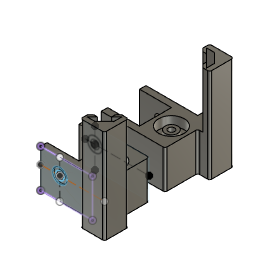
Bed Mount Lighted (Autodesk Fusion 360 design; units mm, degrees)
part number: Mount
Autodesk Fusion 360 part; units mm, degrees
sketch "Sketch1" plane through (0, 0, 0) normal (0, 0, 1) x (1, 0, 0) in component "Mount"
  line L0 (20, 14) -> (-20, 14)
  line L1 (-20, 14) -> (-20, -14)
  line L2 (-20, -14) -> (20, -14)
  line L3 (20, -14) -> (20, 14)
  line L4 (20, 14) -> (-20, -14) construction
  line L5 (-20, 14) -> (20, -14) construction
  line L6 (27.5, -6.5) -> (12.5, -6.5)
  line L7 (12.5, -6.5) -> (12.5, -21.5)
  line L8 (12.5, -21.5) -> (27.5, -21.5)
  line L9 (27.5, -21.5) -> (27.5, -6.5)
  line L10 (27.5, -6.5) -> (12.5, -21.5) construction
  line L11 (12.5, -6.5) -> (27.5, -21.5) construction
  circle A0 centre (20, -14) radius 2
  line L12 (-50.6041, 25.2183) -> (52.08, 25.2183) construction
  point P0 (20, -14)
  dimension "d1" = 40
  dimension "d2" = 28
  dimension "d53" = 15
  dimension "d54" = 15
  dimension "d67" = 4
  constraint perpendicular L0 L1
  constraint parallel L0 L2
  constraint parallel L1 L3
  constraint horizontal L0
  constraint coincident L4 origin
  constraint coincident L5 origin
  constraint horizontal L6
  constraint perpendicular L6 L7
  constraint parallel L6 L8
  constraint parallel L7 L9
  constraint coincident L10 P0
  constraint coincident L11 P0
  constraint coincident P0 L2.end
  constraint perpendicular L3 L12
  measures "d1" distance of L1.end P0
  measures "d2" distance of L0.end L1.end
  measures "d53" distance of L7.end L8.end
  measures "d54" distance of L6.end L7.end
  measures "d67" diameter of A0
extrude "Extrude1" add sketch "Sketch1" along normal blind 24 contours L0 L1 L2 L3 L6 L7 | L2 L3 L6 L7 A0 makes body 1 in component "Mount"
extrude "Extrude11" add sketch "Sketch1" along normal blind 59 contours L2 L3 L6 L7 L8 L9 A0 | L2 L3 L6 L7 A0 bodies 1 in component "Mount"
sketch "Sketch1 (2)" plane through (0, 0, 59) normal (0, 0, 1) x (-1, 0, 0)
  line L0 (-27.5, 21.5) -> (-27.5, 6.5)
  line L1 (-27.5, 6.5) -> (-12.5, 6.5)
  line L2 (-12.5, 6.5) -> (-12.5, 21.5)
  line L3 (-12.5, 21.5) -> (-27.5, 21.5)
  line L4 (-12.5, 6.5) -> (-14.5, 6.5)
  line L5 (-14.5, 6.5) -> (-14.5, 15.25)
  line L6 (-14.5, 15.25) -> (-12.5, 15.25)
  line L7 (-12.5, 15.25) -> (-12.5, 6.5)
  line L8 (-12.5, 6.5) -> (-21.25, 6.5)
  line L9 (-21.25, 6.5) -> (-21.25, 8.5)
  line L10 (-21.25, 8.5) -> (-12.5, 8.5)
  line L11 (-12.5, 8.5) -> (-12.5, 6.5)
  line L12 (-14.5, 8.5) -> (-21.25, 8.5)
  line L13 (-21.25, 8.5) -> (-21.25, 15.25)
  line L14 (-21.25, 15.25) -> (-14.5, 15.25)
  line L15 (-14.5, 15.25) -> (-14.5, 8.5)
  line L16 (-12.5, 19.5) -> (-25.5, 6.5)
  line L17 (-14.5, 15.25) -> (-14.5, 17.5)
  line L18 (-21.25, 8.5) -> (-21.25, 10.75)
  line L19 (-14.5, 15.25) -> (-16.75, 15.25)
  line L20 (-21.25, 8.5) -> (-23.5, 8.5)
  line L21 (-27.5, 21.5) -> (-13.5, 21.5)
  line L22 (-13.5, 21.5) -> (-13.5, 18.5)
  line L23 (-13.5, 18.5) -> (-27.5, 18.5)
  line L24 (-27.5, 18.5) -> (-27.5, 21.5)
  line L25 (-27.5, 21.5) -> (-24.5, 21.5)
  line L26 (-24.5, 21.5) -> (-24.5, 7.5)
  line L27 (-24.5, 7.5) -> (-27.5, 7.5)
  line L28 (-27.5, 7.5) -> (-27.5, 21.5)
  circle A0 centre (-20, 14) radius 2
  dimension "d57" = 2
  dimension "d58" = 8.75
  dimension "d59" = 8.75
  dimension "d60" = 2
  dimension "d61" = 2
  dimension "d62" = 2
  dimension "d63" = 3
  dimension "d64" = 3
  constraint horizontal L4
  constraint vertical L5
  constraint horizontal L6
  constraint vertical L7
  constraint coincident L1.end L2.start
  constraint horizontal L8
  constraint vertical L9
  constraint horizontal L10
  constraint vertical L11
  constraint horizontal L12
  constraint vertical L13
  constraint horizontal L14
  constraint vertical L15
  constraint coincident L10 L12.start
  constraint coincident L5 L12.start
  constraint coincident L2 L16.start
  constraint coincident L1 L16.end
  constraint coincident L16 L17.end
  constraint perpendicular L14 L17
  constraint coincident L16 L18.end
  constraint coincident L13 L18.end
  constraint perpendicular L10 L18
  constraint coincident L16 L19.end
  constraint coincident L14 L19.end
  constraint perpendicular L17 L19
  constraint coincident L16 L20.end
  constraint perpendicular L9 L20
  constraint horizontal L21
  constraint vertical L22
  constraint horizontal L23
  constraint vertical L24
  constraint coincident L16 L22.end
  constraint coincident L0.start L3.end
  constraint horizontal L25
  constraint vertical L26
  constraint horizontal L27
  constraint vertical L28
  constraint coincident L16 L26.end
  measures "d57" distance of L1.end L4.end
  measures "d58" distance of L1.end L6.end
  measures "d59" distance of L1.end L8.end
  measures "d60" distance of L1.end L10.end
  measures "d61" distance of L0.end L16.end
  measures "d62" distance of L2.end L16.start
  measures "d63" distance of L0.start L23.end
  measures "d64" distance of L0.start L25.end
extrude "Extrude12" cut sketch "Sketch1 (2)" against normal blind 35 contours L13 L14 L16 L23 L26 A0 | L1 L5 L8 L9 L10 L12 | L5 L10 L12 L13 L14 L15 L16 L18 L19 A0 | L13 L16 A0 | L2 L5 L6 L7 L10 L15 | L14 L16 A0 | L1 L2 L4 L5 L7 L8 L10 L11 | L13 L14 A0 | L13 L14 L16 A0 | L16 A0 bodies 1 in component "Mount"
sketch "Sketch2" plane through (0, 0, 24) normal (0, 0, 1) x (-1, 0, 0) in component "Mount"
  line L0 (-20, -14) -> (20, -14)
  line L1 (20, -14) -> (20, 14)
  line L2 (20, -10) -> (0, -10)
  line L3 (0, -10) -> (0, 10)
  line L4 (0, 10) -> (20, 10)
  line L5 (20, 10) -> (20, -10)
  line L6 (-12.5, 14) -> (-12.5, 15.25)
  line L7 (-21.25, 6.5) -> (-20, 6.5)
  line L8 (-20, 6.5) -> (-20, -14)
  line L9 (20, 14) -> (-12.5, 14)
  circle A0 centre (-20, 14) radius 2
  line L10 (-12.5, 15.25) -> (-16.75, 15.25)
  line L11 (-16.75, 15.25) -> (-13.5, 18.5)
  line L12 (-13.5, 18.5) -> (-24.5, 18.5)
  line L13 (-24.5, 18.5) -> (-24.5, 7.5)
  line L14 (-24.5, 7.5) -> (-21.25, 10.75)
  line L15 (-21.25, 10.75) -> (-21.25, 6.5)
  dimension "d5" = 20
  dimension "d6" = 20
  dimension "d7" = 4
  constraint horizontal L2
  constraint vertical L3
  constraint horizontal L4
  constraint vertical L5
  constraint coincident L1 L2.start
  measures "d5" distance of L2.start L4.end
  measures "d6" distance of L2.start L2.end
  measures "d7" distance of L0 L2
extrude "Extrude2" cut sketch "Sketch2" against normal blind 20 contours L1 L2 L3 L4 L5 bodies 1 in component "Mount"
sketch "Sketch3" plane through (0, -14, 0) normal (0, -1, 0) x (1, 0, 0) in component "Mount"
  line L0 (-20, 24) -> (-20, 0)
  line L1 (-8, 0) -> (-8, 24) construction
  line L2 (-20, 14) -> (20, 14) construction
  circle A0 centre (-8, 14) radius 2.5
  circle A1 centre (-8, 14) radius 4.5
  line L3 (12.5, 0) -> (12.5, 24)
  line L4 (12.5, 24) -> (-20, 24)
  line L5 (-20, 0) -> (12.5, 0)
  dimension "d10" = 12
  dimension "d12" = 5
  dimension "d13" = 9
  constraint coincident L0 L2.start
  constraint coincident L2 A0.centre
  constraint coincident L1 A0.centre
  constraint concentric A0 A1
  measures "d10" distance of L0 L1
  measures "d12" diameter of A0
  measures "d13" diameter of A1
extrude "Extrude4" cut sketch "Sketch3" against normal blind 1 contours A0 | A1 bodies 1 in component "Mount"
extrude "Extrude3" cut sketch "Sketch3" against normal blind 4 contours A0 bodies 1 in component "Mount"
sketch "Sketch4" plane through (0, 14, 0) normal (0, 1, 0) x (-1, 0, 0) in component "Mount"
  line L0 (-20, 0) -> (20, 0)
  line L1 (20, 0) -> (20, 24)
  line L2 (20, 24) -> (-20, 24)
  line L3 (-20, 24) -> (-20, 0)
  line L4 (14, 24) -> (14, 0) construction
  line L5 (20, 14) -> (-20, 14) construction
  circle A0 centre (14, 14) radius 2.5
  circle A1 centre (14, 14) radius 4.5
  dimension "d18" = 10
  dimension "d19" = 6
  dimension "d20" = 5
  dimension "d21" = 9
  constraint coincident L2 L4.start
  constraint coincident L0 L4.end
  constraint perpendicular L0 L4
  constraint coincident L1 L5.start
  constraint coincident L3 L5.end
  constraint perpendicular L3 L5
  constraint coincident L5 A0.centre
  constraint coincident L4 A0.centre
  constraint concentric A0 A1
  measures "d18" distance of L2 L5
  measures "d19" distance of L1 L4
  measures "d20" diameter of A0
  measures "d21" diameter of A1
extrude "Extrude6" cut sketch "Sketch4" against normal blind 1 contours A0 | A1 bodies 1 in component "Mount"
extrude "Extrude5" cut sketch "Sketch4" against normal blind 4 contours A0 bodies 1 in component "Mount"
sketch "Sketch5" plane through (0, 0, 24) normal (0, 0, 1) x (-1, 0, 0) in component "Mount"
  line L0 (0, 10) -> (20, 10)
  line L1 (20, 10) -> (20, 14)
  line L2 (20, 14) -> (-12.5, 14)
  line L3 (-20, 6.5) -> (-20, -14)
  line L4 (-20, -14) -> (20, -14)
  line L5 (20, -10) -> (0, -10)
  line L6 (0, -10) -> (0, 10)
  line L7 (0, -10) -> (-20, -10) construction
  line L8 (0, 10) -> (-20, 10) construction
  line L9 (-20, 10) -> (0, -10) construction
  line L10 (0, 10) -> (-20, -10) construction
  circle A0 centre (-10, 0) radius 8
  circle A1 centre (-10, 0) radius 4
  circle A2 centre (-10, 0) radius 2
  line L11 (-12.5, 14) -> (-12.5, 15.25)
  line L12 (-21.25, 6.5) -> (-20, 6.5)
  line L13 (-12.5, 15.25) -> (-16.75, 15.25)
  line L14 (-16.75, 15.25) -> (-13.5, 18.5)
  line L15 (-13.5, 18.5) -> (-24.5, 18.5)
  line L16 (-24.5, 18.5) -> (-24.5, 7.5)
  line L17 (-24.5, 7.5) -> (-21.25, 10.75)
  line L18 (-21.25, 10.75) -> (-21.25, 6.5)
  line L19 (20, -14) -> (20, -10)
  circle A3 centre (-20, 14) radius 2
  line L20 (-17.7, 18.5) -> (-24.5, 11.7)
  line L21 (-21.25, 10.75) -> (-16.75, 15.25)
  dimension "d26" = 16
  dimension "d27" = 8
  dimension "d28" = 4
  dimension "d69" = 4.2
  dimension "d70" = 4.2
  constraint coincident L5.end L6.start
  constraint coincident L3 L7.end
  constraint perpendicular L3 L7
  constraint coincident L0.start L6.end
  constraint coincident L3 L8.end
  constraint perpendicular L3 L8
  constraint midpoint L10 A0.centre
  constraint concentric A0 A1
  constraint concentric A0 A2
  constraint coincident L15 L20.start
  constraint coincident L16 L20.end
  constraint coincident L17.end L18.start
  constraint coincident L13.end L14.start
  measures "d26" diameter of A0
  measures "d27" diameter of A1
  measures "d28" diameter of A2
  measures "d69" distance of L14.end L20.start
  measures "d70" distance of L16.end L20.end
extrude "Extrude13" cut sketch "Sketch5" against normal blind 10 contours L14 L15 A3 L20 L21 | L16 L17 A3 L20 L21 bodies 1 in component "Mount"
extrude "Extrude7" cut sketch "Sketch5" against normal blind 6 contours A0 | A1 | A2 bodies 1 in component "Mount"
extrude "Extrude8" add sketch "Sketch5" along normal blind 4 from surface at -6 contours A1 bodies 1 in component "Mount"
extrude "Extrude9" cut sketch "Sketch5" against normal blind 18.3 contours A2 bodies 1 in component "Mount"
sketch "Sketch6" plane through (0, 0, 0) normal (0, 0, -1) x (1, 0, 0) in component "Mount"
  line L0 (-20, -14) -> (20, -14)
  line L1 (20, -14) -> (20, 6.5)
  line L2 (12.5, 14) -> (-20, 14)
  line L3 (-20, 14) -> (-20, -14)
  line L4 (12.8, -1.6166) -> (12.8, 1.6166)
  line L5 (12.8, 1.6166) -> (10, 3.2332)
  line L6 (10, 3.2332) -> (7.2, 1.6166)
  line L7 (7.2, 1.6166) -> (7.2, -1.6166)
  line L8 (7.2, -1.6166) -> (10, -3.2332)
  line L9 (10, -3.2332) -> (12.8, -1.6166)
  line L10 (10, 0) -> (10, 14) construction
  line L11 (20, 6.5) -> (27.5, 6.5)
  line L12 (27.5, 6.5) -> (27.5, 21.5)
  line L13 (27.5, 21.5) -> (12.5, 21.5)
  line L14 (12.5, 21.5) -> (12.5, 14)
  circle A0 centre (20, 14) radius 2
  point P0 (10, 0)
  dimension "d50" = 2.8
  constraint coincident P0 L10.start
  constraint coincident L2 L10.end
  constraint perpendicular L2 L10
  constraint coincident L5.end L10
  measures "d50" distance of P0 L9
extrude "Extrude10" cut sketch "Sketch6" against normal blind 5.5 contours L4 L5 L6 L7 L8 L9 bodies 1 in component "Mount"
fillet "Fillet3" radius 1.25 5 edges at (20, 14, 12) (27.5, -21.5, 29.5) (27.5, -6.5, 29.5) (12.5, -21.5, 29.5) (20, -6.5, 12) on bodies 1 in component "Mount"
chamfer "Chamfer3" distance 2 angle 45 1 edges at (21.25, -6.5, 41.5) measured on face at (24.5833, -6.5, 27.6667) on bodies 1 in component "Mount"
chamfer "Chamfer1" distance 5 angle 45 2 edges at (18.6625, -15.487, 14) (21.487, -12.6625, 14) on bodies 1 in component "Mount"
chamfer "Chamfer2" distance 2 angle 45 1 edges at (12.5, -15.25, 41.5) measured on face at (12.5, -16.5, 8) on bodies 1 in component "Mount"
chamfer "Chamfer4" distance 6 angle 45 1 edges at (24.5, -18.5, 41.5) measured on face at (18.5667, -18.5, 47.3333) on bodies 1 in component "Mount"
ref_plane "WorkPlane1" through (0, 19, 12) normal (0, 1, 0) x (-1, 0, 0) in component "Mount"
mirror "Mirror1" about plane through (0, 19, 12) normal (0, 1, 0) of bodies 1 makes body 2 in component "Mount"
component "Mount" placed x (1, 0, 0) y (0, 1, 0) z (0, 0, 1) at (0, 0, 0)
equation "d55 = 24 mm + 35 mm"
